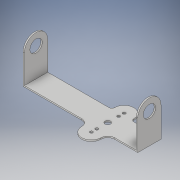
# Autodesk Inventor part: Another Motor Bracket
Saved by Autodesk Inventor 2017 (Build 210142000, 142)
## iProperties
Created: 2017-06-23
Part Number: Another Motor Bracket
Material: Generic
Document SubType Name: Modeling
Designer: Matthew
Density: 1 g/cm^3
Appearance: Default
Author: Matthew
Autodesk Inventor part; units mm, degrees
ref_plane "YZ Plane" through (0, 0, 0) normal (1, 0, 0) x (0, 1, 0)
ref_plane "XZ Plane" through (0, 0, 0) normal (0, 1, 0) x (-1, 0, 0)
ref_plane "XY Plane" through (0, 0, 0) normal (0, 0, 1) x (1, 0, 0)
sketch "Sketch1" plane through (0, 0, 0) normal (1, 0, 0) x (0, 1, 0)
  circle A0 centre (0, 0) radius 14.2875
  line L0 (-66.3768, 26.9875) -> (-66.3768, -26.9875)
  circle A1 centre (0, 0) radius 26.9875
  line L1 (0, 26.9875) -> (-66.3768, 26.9875)
  line L2 (0, -26.9875) -> (-66.3768, -26.9875)
  point P0 (-66.3768, 0)
  dimension "d0" = 28.575
  dimension "d1" = 66.3768
  dimension "d2" = 53.975
  dimension "d3" = 12.7
  constraints: 6 end point, 2 centre point, 2 point on circle, 1 coincident, 1 horizontal, 1 horizontal alignment, 1 midpoint, 1 parallel, 1 vertical
  measures "d0" diameter of A0
  measures "d1" distance from line of point (0, 0) L0
  measures "d2" distance of L0.start L0.end
  measures "d3" radial gap between concentric circles of A0 A1
extrude "Extrusion1" add sketch "Sketch1" along normal blind 3.175
sketch "Sketch2" plane through (0, -66.3768, -26.9875) normal (0, -1, 0) x (1, 0, 0)
  line L0 (0, 0) -> (0, 53.975) projected
  line L1 (0, 53.975) -> (133.35, 53.975)
  line L2 (133.35, 53.975) -> (133.35, 0)
  line L3 (133.35, 0) -> (0, 0)
  line L4 (0, 0) -> (0, 53.975)
  point P0 (0, 26.9875)
  dimension "d6" = 53.975
  dimension "d7" = 133.35
  constraints: 8 end point, 2 parallel, 1 horizontal, 1 perpendicular
  measures "d6" distance of L1.end L2.end
  measures "d7" distance of L2.end L3.end
extrude "Extrusion2" add sketch "Sketch2" along normal blind 3.175
mirror "Mirror1" about plane through (133.35, -66.3768, -26.9875) normal (1, 0, 0)
sketch "Sketch3" plane through (0, -66.3768, -26.9875) normal (0, 1, 0) x (1, 0, 0)
  line L0 (3.175, -53.975) -> (3.175, 0) projected
  line L1 (3.175, -53.975) -> (263.525, -53.975) projected
  line L2 (263.525, -53.975) -> (263.525, 0) projected
  line L3 (263.525, 0) -> (3.175, 0) projected
  circle A0 centre (174.625, -31.745) radius 6.35
  circle A1 centre (174.625, -6.345) radius 3.3528
  circle A2 centre (174.625, 6.355) radius 3.3528
  circle A3 centre (174.625, -57.145) radius 3.3528
  circle A4 centre (174.625, -69.845) radius 3.3528
  arc A5 (152.2222, -69.845) -> (197.0278, -69.845) centre (174.625, -69.845) ccw
  arc A6 (197.0278, 6.355) -> (152.2222, 6.355) centre (174.625, 6.355) ccw
  line L4 (263.525, 0) -> (3.175, 0) projected
  line L5 (3.175, -53.975) -> (263.525, -53.975) projected
  arc A7 (197.0278, 6.355) -> (203.3828, 0) centre (203.3828, 6.355) ccw
  arc A8 (145.8672, 0) -> (152.2222, 6.355) centre (145.8672, 6.355) ccw
  arc A9 (152.2222, -69.845) -> (136.3522, -53.975) centre (136.3522, -69.845) ccw
  arc A10 (212.8978, -53.975) -> (197.0278, -69.845) centre (212.8978, -69.845) ccw
  point P0 (0, -26.9875)
  dimension "d10" = 22.23
  dimension "d11" = 12.7
  dimension "d12" = 47.63
  dimension "d13" = 6.7056
  dimension "d14" = 6.7056
  dimension "d15" = 60.33
  dimension "d16" = 6.7056
  dimension "d17" = 3.17
  dimension "d18" = 6.7056
  dimension "d19" = 15.87
  dimension "d20" = 88.9
  dimension "d21" = 19.05
  dimension "d22" = 19.05
  constraints: 12 point on circle, 11 centre point, 8 tangent, 4 horizontal alignment, 4 point on line, 4 vertical alignment, 2 coincident
  measures "d10" distance from line of L1 A0.centre
  measures "d11" diameter of A0
  measures "d12" distance from line of L1 A1.centre
  measures "d13" diameter of A1
  measures "d14" diameter of A2
  measures "d15" distance from line of L1 A2.centre
  measures "d16" diameter of A3
  measures "d17" distance from line of L1 A3.centre
  measures "d18" diameter of A4
  measures "d19" distance from line of L1 A4.centre
  measures "d20" distance from line of L2 A0.centre
  measures "d21" radial gap between concentric circles of A5 A4
  measures "d22" radial gap between concentric circles of A6 A2
extrude "Extrusion3" add sketch "Sketch3" against normal blind 3.175 contours L0 L3 L2 L1 A3 | L1 A3 A10 A5 A9 | A8 A6 A7 L3 | A3 L1 | L1 A3 | A0 | A1 | A2 | A4
extrude "Extrusion4" cut sketch "Sketch3" against normal blind 3.175 contours A3 L1 | L1 A3 | A0 | A1 | A2 | A4
body "Solid1"
